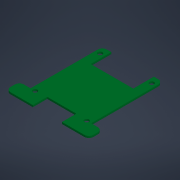
# Autodesk Inventor part: SubBoard
Saved by Autodesk Inventor 2022 (Build 260153000, 153)
## iProperties
Created: 2022-03-28
Part Number: SubBoard
Material: 一般
Document SubType Name: Modeling
Designer: neko2
Density: 1 g/cm^3
Appearance: 基板
Author: neko2
Autodesk Inventor part; units mm, degrees
ref_plane "YZ Plane" through (0, 0, 0) normal (1, 0, 0) x (0, 1, 0)
ref_plane "XZ Plane" through (0, 0, 0) normal (0, 1, 0) x (-1, 0, 0)
ref_plane "XY Plane" through (0, 0, 0) normal (0, 0, 1) x (1, 0, 0)
sketch "スケッチ1" plane through (0, 0, 0) normal (0, 1, 0) x (-1, 0, 0)
  line L0 (-13.5, -15.8718) -> (-13.5, 16.1282)
  circle A0 centre (-11.5, 16.1282) radius 0.8 projected
  line L1 (-13.5, -10.6768) -> (-13.5, 15.3232) projected
  line L2 (-13.5, 16.1282) -> (-13.5, 10.2382) projected
  line L3 (-13.5, 10.2382) -> (-13.5, -3.9818) projected
  line L4 (-13.5, -3.9818) -> (-13.5, -15.8718) projected
  line L5 (-13.5, -15.8718) -> (-9.5, -15.8718) projected
  line L6 (-9.5, -15.8718) -> (-9.5, -9.8718)
  circle A1 centre (-11.5, 16.1282) radius 0.8 projected
  line L7 (-18.5, 22.1282) -> (0, 22.1282)
  line L8 (-13.5, -15.8718) -> (-9.5, -15.8718)
  line L9 (-9.5, -15.8718) -> (-9.5, -9.8718)
  line L10 (-9.5, -6.6718) -> (0, -6.6718)
  line L11 (-9.5, -15.8718) -> (-9.5, -6.6718)
  line L12 (0, 22.1282) -> (0, -6.6718)
  line L13 (13.5, -15.8718) -> (13.5, 16.1282)
  line L14 (13.5, -15.8718) -> (9.5, -15.8718)
  line L15 (18.5, 22.1282) -> (0, 22.1282)
  line L16 (9.5, -6.6718) -> (0, -6.6718)
  line L17 (9.5, -15.8718) -> (9.5, -6.6718)
  circle A2 centre (-11.5, -12.8718) radius 1
  circle A3 centre (-11.5, 16.1282) radius 1
  circle A4 centre (11.5, -12.8718) radius 1
  circle A5 centre (-11.5, 16.1282) radius 1 projected
  circle A6 centre (11.5, 16.1282) radius 1 projected
  circle A7 centre (-11.5, -12.8718) radius 1 projected
  circle A8 centre (11.5, -12.8718) radius 1 projected
  circle A9 centre (0, -12.6718) radius 7.5 projected
  spline S0 degree 3 poles (0, -30.8718) (-3.9797, -30.6573) (-6.3943, -30.6605) (-10.2198, -30.5013) (-11.7409, -30.3574) (-14.0031, -29.6154) (-14.9542, -29.1518) (-16.6972, -27.6417) (-17.3717, -26.7721) (-18.3737, -25.0018) (-18.7365, -24.1111) (-19.2696, -22.239) (-19.4316, -21.261) (-19.5, -20.2718) knots 0 0 0 0 1.195654 1.195654 2.243866 2.243866 2.930767 2.930767 3.539935 3.539935 4.077393 4.077393 4.633359 4.633359 4.633359 4.633359 projected
  spline S1 degree 3 poles (19.5, -20.2718) (19.3569, -22.3429) (18.8278, -24.0013) (17.6447, -26.3968) (16.8969, -27.447) (15.0392, -29.0976) (14.097, -29.571) (12.111, -30.2513) (10.9109, -30.4205) (7.3866, -30.667) (4.5667, -30.6246) (0, -30.8718) knots 0 0 0 0 0.622814 0.622814 1.176012 1.176012 1.714262 1.714262 2.395692 2.395692 3.535201 3.535201 3.535201 3.535201 projected
  line L18 (19.5, -10.8718) -> (19.5, -20.2718) projected
  arc A10 (19.5, -10.8718) -> (18.5, -9.8718) centre (18.5, -10.8718) ccw projected
  line L19 (13.5, -9.8718) -> (18.5, -9.8718) projected
  line L20 (13.5, 16.1282) -> (13.5, -9.8718) projected
  line L21 (18.5, 16.1282) -> (13.5, 16.1282) projected
  arc A11 (18.5, 16.1282) -> (19.5, 17.1282) centre (18.5, 17.1282) ccw projected
  line L22 (19.5, 21.1282) -> (19.5, 17.1282) projected
  arc A12 (19.5, 21.1282) -> (18.5, 22.1282) centre (18.5, 21.1282) ccw projected
  line L23 (-18.5, 22.1282) -> (18.5, 22.1282) projected
  arc A13 (-18.5, 22.1282) -> (-19.5, 21.1282) centre (-18.5, 21.1282) ccw projected
  line L24 (-19.5, 17.1282) -> (-19.5, 21.1282) projected
  arc A14 (-19.5, 17.1282) -> (-18.5, 16.1282) centre (-18.5, 17.1282) ccw projected
  line L25 (-13.5, 16.1282) -> (-18.5, 16.1282) projected
  line L26 (-13.5, -9.8718) -> (-13.5, 16.1282) projected
  line L27 (-18.5, -9.8718) -> (-13.5, -9.8718) projected
  arc A15 (-18.5, -9.8718) -> (-19.5, -10.8718) centre (-18.5, -10.8718) ccw projected
  line L28 (-19.5, -20.2718) -> (-19.5, -10.8718) projected
  circle A16 centre (-11.5, 16.1282) radius 1 projected
  circle A17 centre (11.5, 16.1282) radius 1 projected
  circle A18 centre (-11.5, -12.8718) radius 1 projected
  circle A19 centre (11.5, -12.8718) radius 1 projected
  circle A20 centre (0, -12.6718) radius 7.5 projected
  spline S2 degree 3 poles (0, -30.8718) (-3.9797, -30.6573) (-6.3943, -30.6605) (-10.2198, -30.5013) (-11.7409, -30.3574) (-14.0031, -29.6154) (-14.9542, -29.1518) (-16.6972, -27.6417) (-17.3717, -26.7721) (-18.3737, -25.0018) (-18.7365, -24.1111) (-19.2696, -22.239) (-19.4316, -21.261) (-19.5, -20.2718) knots 0 0 0 0 1.195654 1.195654 2.243866 2.243866 2.930767 2.930767 3.539935 3.539935 4.077393 4.077393 4.633359 4.633359 4.633359 4.633359 projected
  spline S3 degree 3 poles (19.5, -20.2718) (19.3569, -22.3429) (18.8278, -24.0013) (17.6447, -26.3968) (16.8969, -27.447) (15.0392, -29.0976) (14.097, -29.571) (12.111, -30.2513) (10.9109, -30.4205) (7.3866, -30.667) (4.5667, -30.6246) (0, -30.8718) knots 0 0 0 0 0.622814 0.622814 1.176012 1.176012 1.714262 1.714262 2.395692 2.395692 3.535201 3.535201 3.535201 3.535201 projected
  line L29 (19.5, -10.8718) -> (19.5, -20.2718) projected
  arc A21 (19.5, -10.8718) -> (18.5, -9.8718) centre (18.5, -10.8718) ccw projected
  line L30 (13.5, -9.8718) -> (18.5, -9.8718) projected
  line L31 (13.5, 16.1282) -> (13.5, -9.8718) projected
  line L32 (18.5, 16.1282) -> (13.5, 16.1282) projected
  arc A22 (18.5, 16.1282) -> (19.5, 17.1282) centre (18.5, 17.1282) ccw projected
  line L33 (19.5, 21.1282) -> (19.5, 17.1282) projected
  arc A23 (19.5, 21.1282) -> (18.5, 22.1282) centre (18.5, 21.1282) ccw projected
  line L34 (-18.5, 22.1282) -> (18.5, 22.1282) projected
  arc A24 (-18.5, 22.1282) -> (-19.5, 21.1282) centre (-18.5, 21.1282) ccw projected
  line L35 (-19.5, 17.1282) -> (-19.5, 21.1282) projected
  arc A25 (-19.5, 17.1282) -> (-18.5, 16.1282) centre (-18.5, 17.1282) ccw projected
  line L36 (-13.5, 16.1282) -> (-18.5, 16.1282) projected
  line L37 (-13.5, -9.8718) -> (-13.5, 16.1282) projected
  line L38 (-18.5, -9.8718) -> (-13.5, -9.8718) projected
  arc A26 (-18.5, -9.8718) -> (-19.5, -10.8718) centre (-18.5, -10.8718) ccw projected
  line L39 (-19.5, -20.2718) -> (-19.5, -10.8718) projected
  line L40 (1.5, 6.1282) -> (1.5, 0.1282) projected
  line L41 (-1.5, 6.1282) -> (-1.5, 0.1282) projected
  line L42 (1.5, 3.1282) -> (-1.5, 3.1282)
  line L43 (13.5, 16.1282) -> (18.5, 16.1282)
  line L44 (-13.5, 16.1282) -> (-18.5, 16.1282)
  line L45 (-18.5, 16.1282) -> (-18.5, 22.1282)
  line L46 (18.5, 16.1282) -> (18.5, 22.1282)
  circle A27 centre (11.5, 16.1282) radius 1
  point P0 (0, 0)
  point P1 (11.5, 16.1282)
  point P2 (0, 3.1282)
  point P3 (4.3, 10.2382)
  point P4 (0, -5.1718)
  point P5 (0, -5.1718)
  point P6 (4.5, -6.6718)
  point P7 (-4.5, -6.6718)
  dimension "d56" = 29
  dimension "d57" = 2
  dimension "d60" = 6
  constraints: 36 end point, 5 point on line, 5 symmetric about line, 4 centre point, 4 midpoint, 3 equal radius, 3 perpendicular, 3 vertical alignment, 2 coincident, 2 collinear, 2 horizontal, 2 vertical, 1 horizontal alignment, 1 parallel, 1 other
  measures "d56" distance of point (-11.5, 16.128) A2.centre
  measures "d57" diameter of A4
  measures "d60" distance from line of L16 A9.centre
extrude "押し出し1" add sketch "スケッチ1" along normal blind 0.8 contours L0 L25 L45 L7 L12 A9 L10 L11 L6 L5 | A9 L12 L10 | L12 A9 L16 | L12 L15 L46 L21 L13 L14 L17 L16 A9
sketch "スケッチ3" plane through (0, 0.8, 0) normal (0, 1, 0) x (1, 0, 0)
  line L0 (6.4, -15.9282) -> (-6.4, -15.9282)
  line L1 (-6.4, -15.9282) -> (-6.4, -22.1282)
  line L2 (6.4, -22.1282) -> (6.4, -15.9282)
  line L3 (-18.5, -22.1282) -> (18.5, -22.1282) projected
  point P0 (0, -15.9282)
  point P1 (0, -22.1282)
  dimension "d26" = 12.8
  dimension "d27" = 6.2
  constraints: 6 end point, 2 midpoint, 2 perpendicular, 2 point on line, 1 parallel, 1 vertical alignment
  measures "d26" distance of L0.start L0.end
  measures "d27" distance of L0.end L1.end
extrude "押し出し3" cut sketch "スケッチ3" against normal through all
fillet "フィレット1" radius 2 6 edges at (13.5, 0.4, -15.8718) (-13.5, 0.4, -15.8718) (-18.5, 0.4, 16.1282) (-18.5, 0.4, 22.1282) (18.5, 0.4, 22.1282) (18.5, 0.4, 16.1282)
